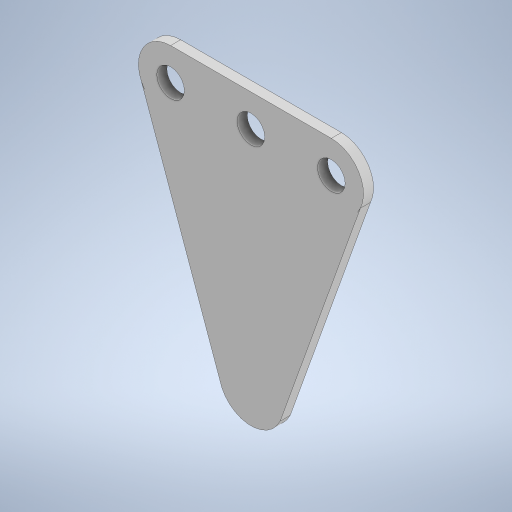
# Autodesk Inventor part: Wing poly short
Saved by Autodesk Inventor 2023 (Build 270158000, 158)
## iProperties
Created: 2024-01-16
Part Number: Wing poly short
Material: Generic
Document SubType Name: Modeling
Designer: Robodox
Density: 1 g/cm^3
Appearance: Default
Author: Robodox
Autodesk Inventor part; units mm, degrees
ref_plane "YZ Plane" through (0, 0, 0) normal (1, 0, 0) x (0, 1, 0)
ref_plane "XZ Plane" through (0, 0, 0) normal (0, 1, 0) x (-1, 0, 0)
ref_plane "XY Plane" through (0, 0, 0) normal (0, 0, 1) x (1, 0, 0)
sketch "Sketch1" plane through (0, 0, 0) normal (0, 0, 1) x (1, 0, 0)
  circle A0 centre (14.1019, 6.1779) radius 2.1844
  circle A1 centre (1.4019, 6.1779) radius 2.1844
  circle A2 centre (-11.2981, 6.1779) radius 2.1844
  circle A3 centre (-23.9981, 6.1779) radius 2.1844
  line L0 (-11.2981, 6.1779) -> (1.4019, 6.1779)
  line L1 (1.4019, 6.1779) -> (14.1019, 6.1779)
  circle A4 centre (-11.2981, 6.1779) radius 5.08
  circle A5 centre (1.4019, 6.1779) radius 5.08
  circle A6 centre (14.1019, 6.1779) radius 5.08
  line L2 (-11.2981, 11.2579) -> (1.4019, 11.2579)
  line L3 (1.4019, 11.2579) -> (14.1019, 11.2579)
  line L4 (1.4019, 6.1779) -> (1.4019, -15.4121)
  circle A7 centre (1.4019, -15.4121) radius 5.08
  circle A8 centre (1.4019, -15.4121) radius 2.1844
  line L5 (-15.8845, 3.9935) -> (-15.4357, 3.2305)
  line L6 (18.2394, 3.2305) -> (18.6882, 3.9935)
  circle A9 centre (1.4019, -29.3531) radius 5.08
  line L7 (-15.8845, 3.9935) -> (-3.2071, -31.4893)
  line L8 (-15.8845, 3.9935) -> (18.6882, 3.9935)
  line L9 (-3.2071, -31.4893) -> (6.0109, -31.4893)
  line L10 (18.6882, 3.9935) -> (6.0109, -31.4893)
  point P0 (0, 0)
  point P1 (0, 0)
  point P2 (5.9211, -31.6732)
  dimension "d1" = 10.16
  dimension "d0" = 10.16
  dimension "d2" = 10.16
  dimension "d3" = 21.59
  dimension "d4" = 10.16
  dimension "d5" = 4.3688
  dimension "d6" = 4.3688
  dimension "d7" = 10.16
  constraints: 22 end point, 9 centre point, 9 point on circle, 5 coincident, 4 horizontal, 1 collinear, 1 point on line, 1 vertical, 1 vertical alignment, 2 other
  measures "d0" diameter of A4
  measures "d2" diameter of A6
  measures "d3" distance of L4.start L4.end
  measures "d4" diameter of A7
  measures "d5" diameter of A0
  measures "d6" diameter of A8
  measures "d7" diameter of A9
extrude "Extrusion1" add sketch "Sketch1" along normal blind 1.5875 contours A0 L1 A6 L8 | A0 L8 A6 L1 | L8 L6 A6 | A6 L8 A5 L1 | L1 A5 L3 A6 | A8 | A7 | A6 L10 A9 L7 A4 L8 A5 | A5 L8 A1 L1 | L1 A1 L0 A5 | A5 L4 L8 | L10 L9 L7 A9 | A5 L0 A4 L2 | A5 L8 L4 | L8 A5 L0 A1 | A9 L9 | A5 L8 A4 L0 | A4 L0 A2 L8 | A4 L8 A2 L0 | L8 A4 L5
body "Solid1"
